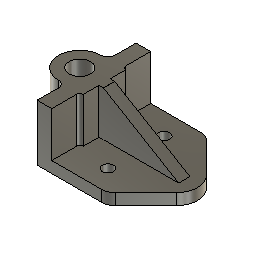
A3 (Autodesk Fusion 360 design; units mm, degrees)
Autodesk Fusion 360 part; units mm, degrees
sketch "Sketch1" plane through (0, 0, 0) normal (0, 0, 1) x (1, 0, 0)
  circle A0 centre (-43, 0) radius 19
  circle A1 centre (-43, 0) radius 9.5
  line L0 (-37, 44) -> (-37, 18.0278)
  line L1 (-37, -44) -> (-37, -18.0278)
  line L2 (-37, -44) -> (43, -44)
  line L3 (-37, 44) -> (43, 44)
  line L4 (-37, 44) -> (-24, 44)
  line L5 (-24, 0) -> (-21, 0)
  line L6 (-21, 19) -> (-24, 19)
  line L7 (-21, -19) -> (-24, -19)
  line L8 (-24, 19) -> (-24, 44)
  line L9 (-24, -19) -> (-24, -44)
  line L10 (-21, 0) -> (-17, 0)
  line L11 (-17, 0) -> (-17, 5)
  line L12 (-17, 0) -> (-17, -5)
  line L13 (-17, 5) -> (-21, 5)
  line L14 (-17, -5) -> (-21, -5)
  line L15 (-21, -5) -> (-21, -19)
  line L16 (-21, 5) -> (-21, 19)
  circle A2 centre (7, 25) radius 5
  circle A3 centre (7, -25) radius 5
  line L17 (43, 44) -> (62, 44)
  line L18 (62, 44) -> (62, -44)
  line L19 (43, -44) -> (62, -44)
  dimension "d8" = 13
  dimension "d21" = 19
  dimension "d22" = 88
  constraint concentric A0 A1
  constraint coincident A0 L0.end
  constraint coincident A0 L1.end
  constraint perpendicular L0 L4
  constraint perpendicular L3 L8
  constraint coincident L2 L9.end
  constraint perpendicular L2 L9
  constraint perpendicular L10 L11
  constraint perpendicular L10 L12
  constraint perpendicular L14 L15
  constraint perpendicular L6 L16
  constraint perpendicular L17 L18
  measures "d8" distance of L0.start L4.end
  measures "d21" distance of L3.end L17.end
  measures "d22" distance of L17.end L18.end
extrude "Extrude1" add sketch "Sketch1" along normal blind 50 contours A0 | A0 L1 L2 L5 L7 L9 L10 L12 L14 L15 | A0 L0 L3 L4 L5 L6 L8 L10 L11 L13 L16
extrude "Extrude2" add sketch "Sketch1" along normal blind 10 contours L2 L3 L6 L7 L8 L9 L11 L12 L13 L14 L15 L16 L17 L18 L19
chamfer "Chamfer1" distance 36.5 angle 45 2 edges at (62, -44, 5) (62, 44, 5)
fillet "Fillet1" radius 19 2 edges at (62, -7.5, 5) (62, 7.5, 5)
fillet "Fillet2" radius 13 1 edges at (25.5, -44, 5)
fillet "Fillet3" radius 13 1 edges at (25.5, 44, 5)
fillet "Fillet4" radius 3 1 edges at (-24, -19, 30)
fillet "Fillet5" radius 3 1 edges at (-24, 19, 30)
fillet "Fillet6" radius 6 1 edges at (-37, 18.0278, 25)
fillet "Fillet7" radius 6 1 edges at (-37, -18.0278, 25)
sketch "Sketch2" plane through (0, 0, 0) normal (0, 1, 0) x (1, 0, 0)
  line L0 (-17.1305, -49.9822) -> (-17.1305, -10.123)
  line L1 (-17.1305, -10.123) -> (49.8695, -10.123)
  line L2 (-17.1305, -49.9822) -> (49.8695, -10.123)
  dimension "d42" = 67
  constraint vertical L0
  constraint perpendicular L0 L1
  measures "d42" distance of L0.end L1.end
extrude "Extrude3" add sketch "Sketch2" along normal mid plane 10
